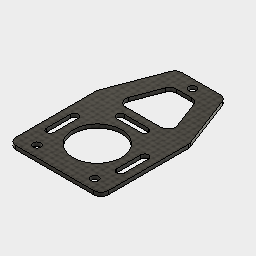
Camera Mounting Plate (Autodesk Fusion 360 design; units mm, degrees)
Autodesk Fusion 360 part; units mm, degrees
note: some values were not read from the file. Set by a fixed rule: which sketch regions a step uses.
sketch "Sketch1" plane through (0, 0, 0) normal (0, 1, 0) x (1, 0, 0)
  circle A0 centre (-12, 0) radius 1.55
  circle A1 centre (12, 0) radius 1.55
  circle A2 centre (0, 13) radius 10
  line L0 (16.1, 13) -> (16.1, 18)
  line L1 (16.1, 13) -> (16.1, 8)
  line L2 (-16.1, 13) -> (-16.1, 18)
  line L3 (-16.1, 13) -> (-16.1, 8)
  line L4 (-13, 13) -> (-13, 18)
  line L5 (-13, 18) -> (-13, 13)
  line L6 (-13, 13) -> (-13, 8)
  line L7 (13, 13) -> (13, 18)
  line L8 (13, 13) -> (13, 8)
  arc A3 (-13, 18) -> (-16.1, 18) centre (-14.55, 18) ccw
  arc A4 (-16.1, 8) -> (-13, 8) centre (-14.55, 8) ccw
  arc A5 (16.1, 18) -> (13, 18) centre (14.55, 18) ccw
  arc A6 (13, 8) -> (16.1, 8) centre (14.55, 8) ccw
  line L9 (0, 29.1) -> (5, 29.1)
  line L10 (0, 29.1) -> (-5, 29.1)
  line L11 (0, 26) -> (5, 26)
  line L12 (5, 26) -> (0, 26)
  line L13 (0, 26) -> (-5, 26)
  arc A7 (-5, 29.1) -> (-5, 26) centre (-5, 27.55) ccw
  arc A8 (5, 26) -> (5, 29.1) centre (5, 27.55) ccw
  line L14 (12, -4.55) -> (16.1, -4.55)
  line L15 (19.1, -1.55) -> (19.1, 13)
  line L16 (-19.1, 13) -> (-19.1, -1.55)
  line L17 (-16.1, -4.55) -> (12, -4.55)
  arc A9 (16.1, -4.55) -> (19.1, -1.55) centre (16.1, -1.55) ccw
  arc A10 (-19.1, -1.55) -> (-16.1, -4.55) centre (-16.1, -1.55) ccw
  circle A11 centre (0, 52.45) radius 1.55
  line L18 (0, 55.95) -> (-7.9306, 55.95)
  line L19 (-19.1, 13) -> (-19.1, 31.4493)
  line L20 (19.1, 13) -> (19.1, 31.4493)
  line L21 (0, 55.95) -> (7.9306, 55.95)
  line L22 (10.735, 54.0156) -> (18.9044, 32.5148)
  line L23 (-10.735, 54.0156) -> (-18.9044, 32.5148)
  line L24 (0, 48.95) -> (3.1021, 48.95)
  line L25 (0, 48.95) -> (-3.1021, 48.95)
  line L26 (7.2626, 32) -> (-7.2626, 32)
  line L27 (10.067, 36.0656) -> (5.9065, 47.0156)
  line L28 (-10.067, 36.0656) -> (-5.9065, 47.0156)
  arc A12 (-10.067, 36.0656) -> (-7.2626, 32) centre (-7.2626, 35) ccw
  arc A13 (7.2626, 32) -> (10.067, 36.0656) centre (7.2626, 35) ccw
  arc A14 (5.9065, 47.0156) -> (3.1021, 48.95) centre (3.1021, 45.95) ccw
  arc A15 (-3.1021, 48.95) -> (-5.9065, 47.0156) centre (-3.1021, 45.95) ccw
  arc A16 (-18.9044, 32.5148) -> (-19.1, 31.4493) centre (-16.1, 31.4493) ccw
  arc A17 (19.1, 31.4493) -> (18.9044, 32.5148) centre (16.1, 31.4493) ccw
  arc A18 (10.735, 54.0156) -> (7.9306, 55.95) centre (7.9306, 52.95) ccw
  arc A19 (-7.9306, 55.95) -> (-10.735, 54.0156) centre (-7.9306, 52.95) ccw
  point P0 (-10, 55.95)
  point P1 (10, 55.95)
extrude "Extrude1" add sketch "Sketch1" along normal blind 1.5
